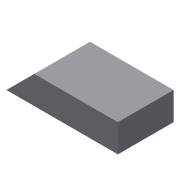
# Autodesk Inventor part: chutebracketv2
Saved by Autodesk Inventor 2015 (Build 190159000, 159)
## iProperties
Created: 2015-03-13
Part Number: chutebracketv2
Material: Generic
Document SubType Name: Modeling
Designer: Jaden
Density: 1 g/cm^3
Appearance: Default
Author: Jaden
Autodesk Inventor part; units mm, degrees
ref_plane "YZ Plane" through (0, 0, 0) normal (1, 0, 0) x (0, 1, 0)
ref_plane "XZ Plane" through (0, 0, 0) normal (0, 1, 0) x (-1, 0, 0)
ref_plane "XY Plane" through (0, 0, 0) normal (0, 0, 1) x (1, 0, 0)
sketch "Sketch1" plane through (0, 0, 0) normal (0, 0, 1) x (1, 0, 0)
  line L0 (0, 0) -> (12.7, 0)
  line L1 (12.7, 0) -> (12.7, 3.175)
  line L2 (0, 0) -> (3.9751, 0) construction
  line L3 (0, 0) -> (3.175, 3.175)
  line L4 (0, 0) -> (4.4901, 0) construction
  line L5 (3.175, 3.175) -> (12.7, 3.175)
  dimension "d0" = 12.7
  dimension "d1" = 3.175
  dimension "d4" = 45
  constraints: 12 end point, 3 horizontal, 1 equal length, 1 perpendicular
  measures "d0" distance of L0.start L0.end
  measures "d1" distance of L0.end L1.end
  measures "d4" angle of L4 L3
extrude "Extrusion2" add sketch "Sketch1" along normal blind 6.35
body "Solid2"
